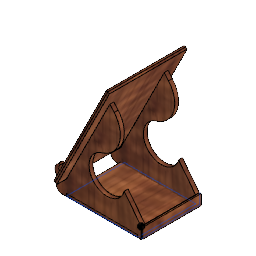
anu v1 (Autodesk Fusion 360 design; units mm, degrees)
Autodesk Fusion 360 part; units mm, degrees
sketch "Sketch1" plane through (0, 0, 0) normal (0, 1, 0) x (1, 0, 0) in component "Component"
sketch "Sketch2" plane through (0, 0, 0) normal (0, 1, 0) x (1, 0, 0) in component "Component"
  line L0 (0, 0) -> (-101.3691, 0)
  line L1 (-101.3691, 0) -> (0, 0)
  line L2 (0, -14.7429) -> (0, 0)
  line L3 (-101.3691, -14.7429) -> (0, -14.7429)
  arc A0 (-101.3691, 0) -> (-101.3691, -14.7429) centre (-101.3691, -7.3714) ccw
  arc A1 (-101.3691, -14.7429) -> (-104.9727, -32.1878) centre (-101.3691, -23.8375) ccw
  line L4 (-39.9142, -129.9008) -> (-95.2219, -19.9874)
  line L5 (-95.2219, -19.9874) -> (-39.9142, -129.9008)
  line L6 (-39.9142, -129.9008) -> (-34.437, -123.5703)
  arc A2 (-34.437, -123.5703) -> (-49.9728, -71.1678) centre (-58.9742, -102.3407) ccw
  arc A3 (-21.6011, -42.7975) -> (-49.9728, -71.1678) centre (-43.616, -49.1533) ccw
  line L7 (-21.6011, -42.7975) -> (0, -14.7429)
  arc A4 (-104.9727, -32.1878) -> (-103.7907, -30.6634) centre (-104.578, -31.2733) ccw
  arc A5 (-95.2219, -19.9874) -> (-103.7907, -30.6634) centre (-98.2261, -26.3529) ccw
  constraint coincident L0.start L1.end
  constraint horizontal L0
  constraint perpendicular L0 L2
  constraint perpendicular L2 L3
  constraint tangent L0 A0
  constraint tangent L3 A0
  constraint tangent L3 A1
  constraint parallel L4 L5
  constraint tangent L6 A2
  constraint tangent A2 A3
  constraint tangent A1 A4
  constraint tangent A4 A5
extrude "Extrude1" add sketch "Sketch2" along normal blind 5 makes body 1 in component "Component"
copy_body "CopyPasteBodies1" bodies 1 makes body 2 in component "Component"
move_body "Move1" bodies 2 to x (1, 0, 0) y (0, 1, 0) z (0, 0, 1) at (0, 69.491, 0.2381) in component "Component"
sketch "Sketch1 (2)" plane through (0, 0, 0) normal (1, 0, 0) x (0, 1, 0) in component "Component'"
  line L0 (-10, 145.7) -> (89.0212, 145.7)
  line L1 (89.0212, 145.7) -> (89.0212, -4.3)
  line L2 (89.0212, -4.3) -> (-10, -4.3)
  line L3 (-10, -4.3) -> (-10, 145.7)
  dimension "d7" = 150
  constraint horizontal L0
  constraint vertical L1
  constraint horizontal L2
  constraint vertical L3
  measures "d7" distance of L0.start L2.end
sketch "Sketch1 (3)" plane through (0, 0, 0) normal (1, 0, 0) x (0, 1, 0) in component "Component''"
  line L0 (85.1618, 170) -> (-10, 170)
  line L1 (-10, 170) -> (-10, 20)
  line L2 (-10, 20) -> (85.1618, 20)
  line L3 (85.1618, 20) -> (85.1618, 170)
  dimension "d8" = 150
  constraint horizontal L0
  constraint vertical L1
  constraint horizontal L2
  constraint vertical L3
  measures "d8" distance of L0.start L2.end
sketch "Sketch1 (4)" plane through (0, 0, 0) normal (1, 0, 0) x (0, 1, 0) in component "Component'''"
sketch "Sketch2 (2)" plane through (-84.0082, 0, 42.2724) normal (-0.893283, 0, 0.449494) x (0, -1, 0) in component "Component'''"
  line L0 (0, -24.9473) -> (0, 98.097)
  line L1 (0, 98.097) -> (-5, 98.097)
  line L2 (-5, 98.097) -> (-5, -24.9473)
  line L3 (-5, -24.9473) -> (0, -24.9473)
  line L4 (-87.2829, 124.4994) -> (12.3691, 124.4994)
  line L5 (12.3691, 124.4994) -> (12.3691, -25.5006)
  line L6 (12.3691, -25.5006) -> (-87.2829, -25.5006)
  line L7 (-87.2829, -25.5006) -> (-87.2829, 124.4994)
  line L8 (-74.8485, 90.3691) -> (-70.097, 90.3691)
  line L9 (-70.097, 90.3691) -> (-70.097, 65.7476)
  line L10 (-70.097, 65.7476) -> (-74.8485, 65.7476)
  line L11 (-74.8485, 65.7476) -> (-74.8485, 90.3691)
  line L12 (-5, 90.3691) -> (0, 90.3691)
  line L13 (0, 90.3691) -> (0, 65.7476)
  line L14 (0, 65.7476) -> (-5, 65.7476)
  line L15 (-5, 65.7476) -> (-5, 90.3691)
  line L16 (-74.4165, 29.4633) -> (-70, 29.4633)
  line L17 (-70, 29.4633) -> (-70, 10)
  line L18 (-70, 10) -> (-74.4165, 10)
  line L19 (-74.4165, 10) -> (-74.4165, 29.4633)
  line L20 (-5, 29.8953) -> (0, 29.8953)
  line L21 (0, 29.8953) -> (0, 10)
  line L22 (0, 10) -> (-5, 10)
  line L23 (-5, 10) -> (-5, 29.8953)
  dimension "d9" = 150
  constraint horizontal L4
  constraint vertical L5
  constraint horizontal L6
  constraint vertical L7
  constraint horizontal L8
  constraint vertical L9
  constraint horizontal L10
  constraint vertical L11
  constraint horizontal L12
  constraint vertical L13
  constraint horizontal L14
  constraint vertical L15
  constraint coincident L0 L13.end
  constraint coincident L2 L12.start
  constraint horizontal L16
  constraint vertical L17
  constraint horizontal L18
  constraint vertical L19
  constraint horizontal L20
  constraint vertical L21
  constraint horizontal L22
  constraint vertical L23
  constraint coincident L0 L21.end
  constraint coincident L2 L20.start
  measures "d9" distance of L4.start L6.end
extrude "Extrude1'" add sketch "Sketch2 (2)" along normal blind 4.5 separate body contours L0 L2 L3 L22 | L0 L2 L14 L20 | L0 L1 L2 L12 | L4 L5 L6 L7 makes body 3 in component "Component'''"
sketch "Sketch1 (5)" plane through (0, 0, 0) normal (0, 0, 1) x (1, 0, 0) in component "Component''''"
  line L0 (-96.0258, 0.4491) -> (-4.8832, 0.4491)
  line L1 (-4.8832, 0.4491) -> (-4.8832, 74.7455)
  line L2 (-4.8832, 74.7455) -> (-96.0258, 74.7455)
  line L3 (-96.0258, 74.7455) -> (-96.0258, 0.4491)
  constraint horizontal L0
  constraint vertical L1
  constraint horizontal L2
  constraint vertical L3
extrude "Extrude1''" add sketch "Sketch1 (5)" along normal blind 3 separate body makes body 4 in component "Component''''"
sketch "Sketch1 (6)" plane through (0, 0, 0) normal (1, 0, 0) x (0, 1, 0) in component "Component'''''"
  line L0 (0, 14.7429) -> (0, 0)
  line L1 (0, 0) -> (5, 0)
  line L2 (5, 0) -> (5, 14.7429)
  line L3 (5, 14.7429) -> (0, 14.7429)
  line L4 (0, 14.7429) -> (74.9999, 14.7429)
  line L5 (74.9999, 14.7429) -> (74.9999, 1.0648)
  line L6 (74.9999, 1.0648) -> (0, 1.0648)
  line L7 (0, 1.0648) -> (0, 14.7429)
  constraint horizontal L4
  constraint vertical L5
  constraint horizontal L6
  constraint vertical L7
  constraint coincident L0.start L3.end
extrude "Extrude1'''" add sketch "Sketch1 (6)" along normal blind 2 separate body contours L0 L2 L3 L4 L6 L7 | L2 L4 L5 L6 makes body 5 in component "Component'''''"
sketch "Sketch1 (7)" plane through (-88.028, 0, 44.2951) normal (-0.893283, 0, 0.449494) x (0, -1, 0) in component "Component''''''"
  line L0 (0, 65.7476) -> (-5, 65.7476)
  line L1 (-5, 65.7476) -> (-5, 90.3691)
  line L2 (-5, 90.3691) -> (0, 90.3691)
  line L3 (0, 90.3691) -> (0, 65.7476)
  line L4 (0, 10) -> (-5, 10)
  line L5 (-5, 10) -> (-5, 29.8953)
  line L6 (-5, 29.8953) -> (0, 29.8953)
  line L7 (0, 29.8953) -> (0, 10)
  line L8 (-70, 10) -> (-74.4165, 10)
  line L9 (-74.4165, 10) -> (-74.4165, 29.4633)
  line L10 (-74.4165, 29.4633) -> (-70, 29.4633)
  line L11 (-70, 29.4633) -> (-70, 10)
  line L12 (-70.097, 65.7476) -> (-74.8485, 65.7476)
  line L13 (-74.8485, 65.7476) -> (-74.8485, 90.3691)
  line L14 (-74.8485, 90.3691) -> (-70.097, 90.3691)
  line L15 (-70.097, 90.3691) -> (-70.097, 65.7476)
  line L16 (-87.2829, -25.5006) -> (12.3691, -25.5006)
  line L17 (12.3691, -25.5006) -> (12.3691, 124.4994)
  line L18 (12.3691, 124.4994) -> (-87.2829, 124.4994)
  line L19 (-87.2829, 124.4994) -> (-87.2829, -25.5006)
  line L20 (-76.0885, 110) -> (1.6459, 110) construction
  line L21 (1.6459, 110) -> (1.6459, 120) construction
  line L22 (1.6459, 120) -> (-76.0885, 120) construction
  line L23 (-76.0885, 120) -> (-76.0885, 110) construction
  line L24 (-62.2931, 94.6263) -> (-15.8332, 94.6263) construction
  line L25 (-15.8332, 94.6263) -> (-15.8332, 104.6263) construction
  line L26 (-15.8332, 104.6263) -> (-62.2931, 104.6263) construction
  line L27 (-62.2931, 104.6263) -> (-62.2931, 94.6263) construction
  line L28 (-55.1873, 76.3914) -> (-17.0281, 76.3914) construction
  line L29 (-17.0281, 76.3914) -> (-17.0281, 86.3914) construction
  line L30 (-17.0281, 86.3914) -> (-55.1873, 86.3914) construction
  line L31 (-55.1873, 86.3914) -> (-55.1873, 76.3914) construction
  constraint perpendicular L20 L21
  constraint parallel L20 L22
  constraint parallel L21 L23
  constraint perpendicular L24 L25
  constraint parallel L24 L26
  constraint parallel L25 L27
  constraint perpendicular L28 L29
  constraint parallel L28 L30
  constraint parallel L29 L31
extrude "Extrude1''''" add sketch "Sketch1 (7)" against normal blind 2 separate body makes body 6 in component "Component''''''"
sketch "Sketch1 (8)" plane through (-88.028, 0, 44.2951) normal (-0.893283, 0, 0.449494) x (0, -1, 0) in component "Component'''''''"
  line L0 (0, 65.7476) -> (-5, 65.7476)
  line L1 (-5, 65.7476) -> (-5, 90.3691)
  line L2 (-5, 90.3691) -> (0, 90.3691)
  line L3 (0, 90.3691) -> (0, 65.7476)
  line L4 (0, 10) -> (-5, 10)
  line L5 (-5, 10) -> (-5, 29.8953)
  line L6 (-5, 29.8953) -> (0, 29.8953)
  line L7 (0, 29.8953) -> (0, 10)
  line L8 (-70, 10) -> (-74.4165, 10)
  line L9 (-74.4165, 10) -> (-74.4165, 29.4633)
  line L10 (-74.4165, 29.4633) -> (-70, 29.4633)
  line L11 (-70, 29.4633) -> (-70, 10)
  line L12 (-70.097, 65.7476) -> (-74.8485, 65.7476)
  line L13 (-74.8485, 65.7476) -> (-74.8485, 90.3691)
  line L14 (-74.8485, 90.3691) -> (-70.097, 90.3691)
  line L15 (-70.097, 90.3691) -> (-70.097, 65.7476)
  line L16 (-87.2829, -25.5006) -> (12.3691, -25.5006)
  line L17 (12.3691, -25.5006) -> (12.3691, 124.4994)
  line L18 (12.3691, 124.4994) -> (-87.2829, 124.4994)
  line L19 (-87.2829, 124.4994) -> (-87.2829, -25.5006)
  line L20 (-66.2529, 112.2058) -> (-3.8994, 112.2058) construction
  line L21 (-3.8994, 112.2058) -> (-3.8994, 122.2058) construction
  line L22 (-3.8994, 122.2058) -> (-66.2529, 122.2058) construction
  line L23 (-66.2529, 122.2058) -> (-66.2529, 112.2058) construction
  line L24 (-60, 90) -> (-16.8652, 90) construction
  line L25 (-16.8652, 90) -> (-16.8652, 100) construction
  line L26 (-16.8652, 100) -> (-60, 100) construction
  line L27 (-60, 100) -> (-60, 90) construction
  line L28 (-60, 70) -> (-21.8408, 70) construction
  line L29 (-21.8408, 70) -> (-21.8408, 80) construction
  line L30 (-21.8408, 80) -> (-60, 80) construction
  line L31 (-60, 80) -> (-60, 70) construction
  text T0 "Anurag Yadav" font "Arial" height 10 align ink ink in box 0 x 0 at (-66.2529, 112.2058) x (1, 0) y (0, 1) spacing 1 kerned height is em
  text T1 "Redmi 5A" font "Arial" height 10 align ink ink in box 0 x 0 at (-60, 90) x (1, 0) y (0, 1) spacing 1 kerned height is em
  text T2 "2019150" font "Arial" height 10 align ink ink in box 0 x 0 at (-60, 70) x (1, 0) y (0, 1) spacing 1 kerned height is em
  constraint perpendicular L20 L21
  constraint parallel L20 L22
  constraint parallel L21 L23
  constraint perpendicular L24 L25
  constraint parallel L24 L26
  constraint parallel L25 L27
  constraint perpendicular L28 L29
  constraint parallel L28 L30
  constraint parallel L29 L31
extrude "Extrude1'''''" add sketch "Sketch1 (8)" against normal blind 3 separate body text T0 T1 T2 makes body 7 at (-55.1946, 53.6936, 109.5452) makes body 8 at (-55.1946, 25.886, 109.5452) makes body 9 at (-52.5592, 34.3203, 110.3332) makes body 10 at (-45.5439, 59.99, 126.4995) makes body 11 at (-44.4713, 43.1541, 128.6309) makes body 12 at (-44.4713, 18.8084, 128.6309) makes body 13 at (-45.8394, 33.4373, 125.9121) makes body 14 at (-33.5989, 61.4968, 150.2378) makes body 15 at (-33.2967, 49.1531, 148.6136) makes body 16 at (-35.9755, 40.5481, 147.7394) makes body 17 at (-35.3569, 34.9245, 148.9688) makes body 18 at (-35.9755, 20.8997, 147.7394) makes body 19 at (-35.9755, 9.7767, 147.7394) makes body 20 at (-33.5989, 15.0564, 150.2378) makes body 21 at (-33.1446, 25.7449, 151.1407) makes body 22 at (-34.19, 7.9877, 149.0631) makes body 23 at (-34.967, 47.7859, 147.519) makes body 24 at (-34.967, 58.8992, 147.519) makes body 25 at (-44.4618, 26.4158, 130.8745) makes body 26 at (-43.7017, 33.4373, 130.1604) makes body 27 at (-46.3296, 41.4793, 127.1627) makes body 28 at (-46.3369, 50.0095, 127.1481) makes body 29 at (-53.4517, 29.7988, 113.0088) makes body 30 at (-55.0522, 38.7908, 109.8283) makes body 31 at (-52.5592, 45.4433, 110.3332) makes body 32 at (-55.6063, 56.8349, 106.5024) in component "Component'''''''"
component "Component" placed x (1, 0, 0) y (0, 1, 0) z (0, 0, 1) at (0, 0, 0)
component "Component'" placed x (1, 0, 0) y (0, 1, 0) z (0, 0, 1) at (0, 0, 0)
component "Component''" placed x (1, 0, 0) y (0, 1, 0) z (0, 0, 1) at (0, 0, 0)
component "Component'''" placed x (1, 0, 0) y (0, 1, 0) z (0, 0, 1) at (0, 0, 0)
component "Component''''" placed x (1, 0, 0) y (0, 1, 0) z (0, 0, 1) at (0, 0, 0)
component "Component'''''" placed x (1, 0, 0) y (0, 1, 0) z (0, 0, 1) at (0, 0, 0)
component "Component''''''" placed x (1, 0, 0) y (0, 1, 0) z (0, 0, 1) at (0, 0, 0)
component "Component'''''''" placed x (1, 0, 0) y (0, 1, 0) z (0, 0, 1) at (0, 0, 0)
equation "len = 150 mm"
equation "thick = 5 mm"
equation "breath = 70 mm"
equation "p_th = 4.5 mm"
equation "d5 = thick"
equation "d7 = len"
equation "d8 = len"
equation "d9 = len"
equation "d10 = p_th"
